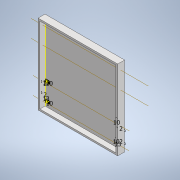
# Autodesk Inventor part: Bottom Base
Saved by Autodesk Inventor 2022 (Build 260153000, 153)
## iProperties
Created: 2022-04-03
Part Number: Bottom Base
Material: Generic
Document SubType Name: Modeling
Designer: Nick
Density: 1 g/cm^3
Appearance: Default
Author: Nick
Autodesk Inventor part; units mm, degrees
ref_plane "YZ Plane" through (0, 0, 0) normal (1, 0, 0) x (0, 1, 0)
ref_plane "XZ Plane" through (0, 0, 0) normal (0, 1, 0) x (-1, 0, 0)
ref_plane "XY Plane" through (0, 0, 0) normal (0, 0, 1) x (1, 0, 0)
sketch "Sketch1" plane through (0, 0, 0) normal (0, 0, 1) x (1, 0, 0)
  line L0 (0, 0) -> (292.1, 0)
  line L1 (292.1, 0) -> (292.1, 292.1)
  line L2 (292.1, 292.1) -> (0, 292.1)
  line L3 (0, 292.1) -> (0, 0)
  dimension "d11" = 292.1
  dimension "d12" = 292.1
  constraints: 8 end point, 2 parallel, 1 horizontal, 1 perpendicular
  measures "d11" distance of L2.end L1.end
  measures "d12" distance of L1.end L0.end
extrude "Extrusion3" add sketch "Sketch1" along normal blind 25.4
sketch "Sketch2" plane through (0, 0, 0) normal (-1, 0, 0) x (0, 0, 1)
  line L0 (25.4, 0) -> (25.4, 292.1) projected
  line L1 (25.4, 0) -> (25.4, 88.9)
  line L2 (25.4, 292.1) -> (25.4, 203.2)
  point P0 (0, 0)
  dimension "d15" = 88.9
  dimension "d16" = 88.9
  constraints: 4 end point, 2 coincident, 2 point on line
  measures "d15" distance of L0.start L1.end
  measures "d16" distance of L0.end L2.end
shell "Shell1" thickness 6.35 removed faces 1 at (97.3667, 194.7333, 25.4)
sketch "Sketch3" plane through (6.35, 6.35, 6.35) normal (1, 0, 0) x (0, 0, -1)
  line L0 (0, 279.4) -> (0, 0) projected
  line L1 (0, 279.4) -> (-19.05, 279.4) projected
  line L2 (-19.05, 0) -> (-19.05, 279.4) projected
  line L3 (0, 0) -> (-19.05, 0) projected
  line L4 (0, 279.4) -> (-19.05, 279.4) projected
  line L5 (-19.05, 260.35) -> (0, 260.35) construction
  line L6 (0, 279.4) -> (0, 0) projected
  line L7 (6.35, 285.75) -> (-19.05, 285.75) projected
  line L8 (6.35, -6.35) -> (-19.05, -6.35) projected
  point P0 (-6.5, 260.35)
  point P1 (-6.5, 196.85)
  point P2 (-6.5, 82.55)
  point P3 (-6.5, 19.05)
  dimension "d20" = 25.4
  dimension "d22" = 88.9
  dimension "d23" = 88.9
  dimension "d24" = 25.4
  dimension "d28" = 6.5
  constraints: 3 point on line, 3 vertical alignment, 2 end point, 1 perpendicular
  measures "d20" distance between parallel lines of L5 L7
  measures "d22" distance from line of L7 point (-6.5, 196.85)
  measures "d23" distance from line of L8 point (-6.5, 82.55)
  measures "d24" distance from line of L8 point (-6.5, 19.05)
  measures "d28" distance from line of L0 point (-6.5, 260.35)
sketch "Sketch5" plane through (6.35, 285.75, 6.35) normal (0, 0, 1) x (1, 0, 0)
  line L0 (277.4, -265.35) -> (264.4, -265.35)
  line L1 (264.4, -265.35) -> (264.4, -255.35)
  line L2 (264.4, -255.35) -> (277.4, -255.35)
  line L3 (277.4, -255.35) -> (277.4, -265.35)
  line L4 (277.4, -201.85) -> (264.4, -201.85)
  line L5 (264.4, -201.85) -> (264.4, -191.85)
  line L6 (264.4, -191.85) -> (277.4, -191.85)
  line L7 (277.4, -191.85) -> (277.4, -201.85)
  line L8 (15, -265.35) -> (2, -265.35)
  line L9 (2, -265.35) -> (2, -255.35)
  line L10 (2, -255.35) -> (15, -255.35)
  line L11 (15, -255.35) -> (15, -265.35)
  line L12 (15, -201.85) -> (2, -201.85)
  line L13 (2, -201.85) -> (2, -191.85)
  line L14 (2, -191.85) -> (15, -191.85)
  line L15 (15, -191.85) -> (15, -201.85)
  line L16 (0, -279.4) -> (0, 0) projected
  line L17 (279.4, 0) -> (279.4, -279.4) projected
  line L18 (4, -264.85) -> (4, -255.85) projected
  line L19 (4, -264.85) -> (9.5, -264.85) projected
  arc A0 (9.5, -264.85) -> (9.5, -255.85) centre (9.5, -260.35) ccw projected
  line L20 (4, -255.85) -> (9.5, -255.85) projected
  circle A1 centre (9.5, -260.35) radius 2 projected
  line L21 (4, -201.35) -> (4, -192.35) projected
  line L22 (4, -201.35) -> (9.5, -201.35) projected
  arc A2 (9.5, -201.35) -> (9.5, -192.35) centre (9.5, -196.85) ccw projected
  line L23 (4, -192.35) -> (9.5, -192.35) projected
  circle A3 centre (9.5, -196.85) radius 2 projected
  line L24 (275.4, -192.35) -> (275.4, -201.35) projected
  line L25 (275.4, -192.35) -> (269.9, -192.35) projected
  arc A4 (269.9, -192.35) -> (269.9, -201.35) centre (269.9, -196.85) ccw projected
  line L26 (275.4, -201.35) -> (269.9, -201.35) projected
  circle A5 centre (269.9, -196.85) radius 2 projected
  line L27 (275.4, -255.85) -> (275.4, -264.85) projected
  line L28 (275.4, -255.85) -> (269.9, -255.85) projected
  arc A6 (269.9, -255.85) -> (269.9, -264.85) centre (269.9, -260.35) ccw projected
  line L29 (275.4, -264.85) -> (269.9, -264.85) projected
  circle A7 centre (269.9, -260.35) radius 2 projected
  point P0 (-6.35, -285.75)
  point P1 (15, -260.35)
  point P2 (264.4, -260.35)
  point P3 (264.4, -196.85)
  point P4 (15, -196.85)
  dimension "d29" = 2
  dimension "d30" = 2
  dimension "d31" = 2
  dimension "d32" = 2
  dimension "d33" = 10
  dimension "d34" = 13
  dimension "d35" = 10
  dimension "d36" = 13
  dimension "d37" = 13
  dimension "d38" = 10
  dimension "d39" = 10
  constraints: 32 end point, 8 parallel, 4 horizontal, 4 horizontal alignment, 4 midpoint, 4 perpendicular, 1 point on line
  measures "d29" distance between parallel lines of L16 L13
  measures "d30" distance between parallel lines of L16 L9
  measures "d31" distance between parallel lines of L17 L3
  measures "d32" distance between parallel lines of L17 L7
  measures "d33" distance of L0.end L1.end
  measures "d34" distance of L0.start L0.end
  measures "d35" distance of L4.end L5.end
  measures "d36" distance of L12.start L12.end
  measures "d37" distance of L9.end L10.end
  measures "d38" distance of L14.end L12.start
  measures "d39" distance of L10.end L8.start
extrude "Extrusion5" cut sketch "Sketch5" against normal blind 1 contours L0 L1 L2 L3 | L4 L5 L6 L7 | L8 L9 L10 L11 | L12 L13 L14 L15 | L18 L20 A0 L19 | A1 | L21 L23 A2 L22 | A3 | L24 L26 A4 L25 | A5 | L27 L29 A6 L28 | A7
sketch "Sketch4" plane through (285.75, 6.35, 6.35) normal (-1, 0, 0) x (0, 0, 1)
  line L0 (0, 0) -> (0, 279.4) projected
  line L1 (0, 0) -> (19.05, 0) projected
  line L2 (19.05, 279.4) -> (19.05, 0) projected
  line L3 (0, 279.4) -> (19.05, 279.4) projected
  line L4 (19.05, 0) -> (0, 21.4113)
  line L5 (0, 0) -> (0, 279.4) projected
  point P0 (-6.35, -6.35)
  point P1 (0, 21.4113)
  dimension "d25" = 41.66
  constraints: 2 end point, 1 point on line
  measures "d25" angle of L4 L0
equation "\"d23\" = d22"
equation "\"d24\" = d20"
body "Solid2"
